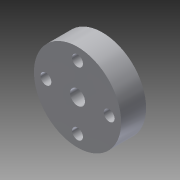
# Autodesk Inventor part: Wheel_MountingHub
Saved by Autodesk Inventor 2013 (Build 170138000, 138)
## iProperties
Created: 2015-07-06
Part Number: Wheel_MountingHub
Material: Aluminum 6061
Document SubType Name: Modeling
Designer: Kyle
Mass: 2.96291 g
Surface Area: 8.96575 cm^2
Volume: 1.09332 cm^3
Density: 2.71 g/cm^3
Author: Kyle
Autodesk Inventor part; units mm, degrees
ref_plane "YZ Plane" through (0, 0, 0) normal (1, 0, 0) x (0, 1, 0)
ref_plane "XZ Plane" through (0, 0, 0) normal (0, 1, 0) x (-1, 0, 0)
ref_plane "XY Plane" through (0, 0, 0) normal (0, 0, 1) x (1, 0, 0)
sketch "Sketch1" plane through (0, 0, 0) normal (0, 0, 1) x (1, 0, 0)
  circle A0 centre (0, 0) radius 8.7503
  circle A1 centre (0, 0) radius 1.4986
  circle A2 centre (-6.35, 0) radius 1.0922
  circle A3 centre (0, 6.35) radius 1.0922
  circle A4 centre (6.35, 0) radius 1.0922
  circle A5 centre (0, -6.35) radius 1.0922
  dimension "d0" = 17.5006
  dimension "d2" = 2.9972
  dimension "d3" = 2.1844
  dimension "d4" = 2.1844
  dimension "d5" = 2.1844
  dimension "d6" = 2.1844
  dimension "d7" = 6.35
  dimension "d8" = 6.35
  dimension "d9" = 6.35
  dimension "d10" = 6.35
  constraints: 6 centre point, 2 coincident
  measures "d0" diameter of A0
  measures "d2" diameter of A1
  measures "d3" diameter of A2
  measures "d4" diameter of A3
  measures "d5" diameter of A4
  measures "d6" diameter of A5
  measures "d7" distance of A4.centre point (0, 0)
  measures "d8" distance of A5.centre point (0, 0)
  measures "d9" distance of A2.centre point (0, 0)
  measures "d10" distance of point (0, 0) A3.centre
extrude "Extrusion1" add sketch "Sketch1" along normal blind 5.0038
body "Solid1"
